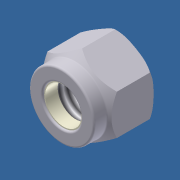
# Autodesk Inventor part: HW-00026
Saved by Autodesk Inventor 2012 (Build 160160000, 160)
## iProperties
Created: 2008-10-27
Part Number: HW-00026
Material: Steel
Description: Nut, Nylock 3/8-16 Zinc Plate
Document SubType Name: Modeling
Designer: firstuser
Mass: 10.5464 g
Surface Area: 10.44 cm^2
Volume: 1.3435 cm^3
Density: 7.85 g/cm^3
Title: Nut, Nylock 3/8-16 Zinc Plate
Author: firstuser
Autodesk Inventor part; units mm, degrees
ref_plane "YZ Plane" through (0, 0, 0) normal (1, 0, 0) x (0, 1, 0)
ref_plane "XZ Plane" through (0, 0, 0) normal (0, 1, 0) x (-1, 0, 0)
ref_plane "XY Plane" through (0, 0, 0) normal (0, 0, 1) x (1, 0, 0)
sketch "Sketch1" plane through (0, 0, 0) normal (0, 0, 1) x (1, 0, 0)
  line L0 (0, 8.1389) -> (7.0485, 4.0695)
  line L1 (7.0485, 4.0695) -> (7.0485, -4.0695)
  line L2 (7.0485, -4.0695) -> (0, -8.1389)
  line L3 (0, -8.1389) -> (-7.0485, -4.0695)
  line L4 (-7.0485, -4.0695) -> (-7.0485, 4.0695)
  line L5 (-7.0485, 4.0695) -> (0, 8.1389)
  line L6 (0, 11.3945) -> (0, -11.3945) projected
  line L7 (-9.8679, 0) -> (9.8679, 0) projected
  point P0 (0, 0)
  dimension "d0" = 14.097
  constraints: 12 end point, 2 midpoint, 1 vertical, 13 other
  measures "d0" distance between parallel lines of L1 L4
extrude "Extrusion1" add sketch "Sketch1" along normal blind 11.6332
sketch "Sketch2" plane through (0, 0, 0) normal (1, 0, 0) x (0, 1, 0)
  line L0 (8.1389, 0) -> (8.1389, 11.6332) projected
  line L1 (4.0695, 11.6332) -> (-4.0695, 11.6332) projected
  line L2 (8.1389, 11.6332) -> (4.0695, 11.6332) projected
  line L3 (4.0695, 11.6332) -> (8.1389, 11.6332) projected
  line L4 (-4.0695, 11.6332) -> (4.0695, 11.6332) projected
  line L5 (-8.1389, 11.6332) -> (-4.0695, 11.6332) projected
  line L6 (-4.0695, 11.6332) -> (-8.1389, 11.6332) projected
  line L7 (8.1389, 7.4422) -> (6.5913, 8.9898)
  line L8 (6.5913, 8.9898) -> (6.5913, 11.6332)
  line L9 (8.1389, 11.6332) -> (8.1389, 7.4422)
  line L10 (6.223, 11.2522) -> (3.683, 11.2522)
  line L11 (3.683, 11.2522) -> (3.683, 8.7122)
  line L12 (3.683, 8.7122) -> (6.223, 8.7122)
  line L13 (6.223, 8.7122) -> (6.223, 11.2522)
  line L14 (0, 18.0282) -> (0, -3.0895) projected
  arc A0 (7.0485, 0) -> (8.1389, 0.762) centre (6.1895, 2.3903) ccw
  line L15 (8.1389, 0) -> (4.0695, 0) projected
  line L16 (7.0485, 0) -> (8.1389, 0)
  line L17 (8.1389, 0.762) -> (8.1389, 0)
  dimension "d3" = 4.191
  dimension "d4" = 45
  dimension "d5" = 6.5913
  dimension "d6" = 3.683
  dimension "d7" = 0.381
  dimension "d8" = 2.54
  dimension "d9" = 2.54
  dimension "d11" = 7.0485
  dimension "d12" = 0.762
  dimension "d13" = 2.54
  constraints: 18 end point, 4 point on line, 3 perpendicular, 2 collinear, 2 parallel, 2 point on circle, 1 centre point, 1 horizontal
  measures "d3" distance of L0.end L7.start
  measures "d4" angle of L9 L7
  measures "d5" distance between parallel lines of L14 L8
  measures "d6" distance between parallel lines of L11 L14
  measures "d7" distance between parallel lines of L10 L2
  measures "d8" distance between parallel lines of L12 L10
  measures "d9" distance of L11.end L12.end
  measures "d11" distance from line of L14 L16.start
  measures "d12" distance of L17.start L0.start
  measures "d13" radius of A0
revolve "Revolution1" cut sketch "Sketch2" angle 360 about axis through (0, 0, 0) along (0, 0, -1) contours L7 L8 L2 L0
revolve "Revolution2" cut sketch "Sketch2" angle 360 about axis through (0, 0, 0) along (0, 0, -1) contours L15 A0 L0
hole "Hole1" at (0, 0, 11.6332) direction (0, 0, -1) diameter 7.7978 end through all thread size "3/8-16 UNC" class "2B" standard "ANSI Unified Screw Threads"
fillet "Fillet1" radius 0.381 3 edges at (0, -6.5913, 8.9898) (0, -6.5913, 11.6332) (0, 3.8989, 11.6332)
revolve "Revolution3" add sketch "Sketch2" angle 360 about axis through (0, 0, 0) along (0, 0, -1) contours L13 L12 L11 L10
body "Solid1"
